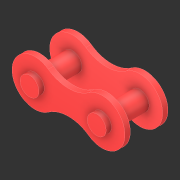
# Autodesk Inventor part: Outer Chain
Saved by Autodesk Inventor 2019 (Build 230136000, 136)
## iProperties
Created: 2020-06-03
Part Number: Outer Chain
Material: Generic
Document SubType Name: Modeling
Designer: 18186
Density: 1 g/cm^3
Appearance: LED - Red On
Author: 18186
Autodesk Inventor part; units mm, degrees
ref_plane "YZ Plane" through (0, 0, 0) normal (1, 0, 0) x (0, 1, 0)
sketch "Sketch1" plane through (0, 0, 0) normal (0, 0, 1) x (1, 0, 0)
  arc A0 (-3.7827, 3.4604) -> (-3.7827, -3.4604) centre (-6.25, 0) ccw
  arc A1 (-3.7827, 3.4604) -> (3.7827, 3.4604) centre (0, 8.7656) ccw
  arc A2 (3.7827, -3.4604) -> (-3.7827, -3.4604) centre (0, -8.7656) ccw
  arc A3 (3.7827, -3.4604) -> (3.7827, 3.4604) centre (6.25, 0) ccw
  line L0 (0, 0) -> (0, 4.5286) construction
  circle A4 centre (-6.25, 0) radius 1.75
  circle A5 centre (6.25, 0) radius 1.75
  point P0 (0, 2.25)
  point P1 (0, -2.25)
  dimension "d0" = 4.5
  dimension "d2" = 8.5
  dimension "d4" = 8.5
  dimension "d5" = 12.5
  dimension "d6" = 3.5
  dimension "d7" = 3.5
  constraints: 10 point on circle, 6 centre point, 4 horizontal alignment, 2 coincident, 2 end point, 2 tangent, 2 vertical alignment, 1 symmetric about line, 1 vertical
  measures "d0" distance of point (0, -2.25) point (0, 2.25)
  measures "d2" diameter of A0
  measures "d4" diameter of A3
  measures "d5" distance of A3.centre A0.centre
  measures "d6" diameter of A4
  measures "d7" diameter of A5
extrude "Extrusion1" add sketch "Sketch1" against normal blind 1
extrude "Extrusion2" add sketch "Sketch1" against normal blind 2 contours A4 | A5
extrude "Extrusion3" add sketch "Sketch1" along normal blind 6 contours A4 | A5
ref_plane "Work Plane1" through (0, 0, 3) normal (0, 0, 1) x (1, 0, 0)
mirror "Mirror1" about plane through (0, 0, 3) normal (0, 0, 1) of "Extrusion1", "Extrusion2"
ref_plane "Work Plane2" through (0, -8.7656, 3) normal (0, 0, 1) x (1, 0, 0)
equation "\"d4\" = d2"
equation "\"d7\" = d6"
body "Solid1"
